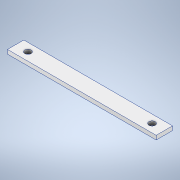
# Autodesk Inventor part: lock ring 1 supp
Saved by Autodesk Inventor 2021 (Build 250183000, 183)
## iProperties
Created: 2021-03-30
Part Number: lock ring 1 supp
Material: Aluminum 6061
Document SubType Name: Modeling
Designer: Work
Density: 2.7 g/cm^3
Appearance: Aluminum - Flat
Mass: 12.2426 g
Surface Area: 37.6973 cm^2
Volume: 4.53429 cm^3
Author: Work
Autodesk Inventor part; units mm, degrees
ref_plane "YZ Plane" through (0, 0, 0) normal (1, 0, 0) x (0, 1, 0)
ref_plane "XZ Plane" through (0, 0, 0) normal (0, 1, 0) x (-1, 0, 0)
ref_plane "XY Plane" through (0, 0, 0) normal (0, 0, 1) x (1, 0, 0)
sketch "Sketch2" plane through (0, 0, 0) normal (0, 1, 0) x (-1, 0, 0)
  line L0 (0, 0) -> (-115.5161, 0)
  line L1 (-115.5161, 0) -> (-115.5161, -12.7)
  line L2 (-115.5161, -12.7) -> (0, -12.7)
  line L3 (0, -12.7) -> (0, 0)
  line L4 (0, -6.35) -> (-115.5161, -6.35)
  point P0 (-9.525, -6.35)
  point P1 (-105.9911, -6.35)
  dimension "d12" = 12.7
  dimension "d13" = 9.525
  dimension "d14" = 9.525
  dimension "d15" = 96.4661
  constraints: 10 end point, 2 midpoint, 2 parallel, 2 point on line, 1 horizontal, 1 perpendicular
  measures "d12" distance of L2.end L0.start
  measures "d13" distance from line of L3 point (-9.525, -6.35)
  measures "d14" distance from line of L1 point (-105.991, -6.35)
  measures "d15" distance of point (-105.991, -6.35) point (-9.525, -6.35)
extrude "Extrusion2" add sketch "Sketch2" along normal blind 3.175
hole "Hole2" at (9.525, 0, -6.35) at (105.9911, 0, -6.35) direction (0, 1, 0) diameter 4.9784 end through all clearance for "Flat Head Machine Screw (82)" size "#10" standard "Ansi Unified Screw Threads"
equation "\"d15\" = ringDiam"
equation "\"height\" = 203.2"
equation "\"thickness\" = 12.7"
equation "\"shaftDiam\" = 6.35"
equation "\"shaftSpace\" = 1.5875"
equation "\"stageSpace\" = 2.54"
equation "\"stageAngle\" = 15deg"
equation "\"bearingDiam\" = 9.5504"
equation "\"FlangeDiam\" = 12.7"
equation "\"FlangeDepth\" = 1.5875"
equation "\"smallFilet\" = 0.39687"
equation "\"ringDiam\" = 96.46608"
equation "\"stockHeight\" = 50.8"
equation "\"stockWidth\" = 76.2"
equation "\"stockRad\" = 9.525"
equation "\"stockGuage\" = 3.175"
equation "\"groundActu\" = 304.8"
equation "\"baseWidth\" = 1066.8"
equation "\"baseDepth\" = 254"
equation "\"capThickness\" = 3.175"
equation "\"sup1Len\" = 660.4"
equation "\"sup1Ang\" = 22.619865deg"
equation "\"sup2Len\" = 2079.37366"
equation "\"sup2Ang\" = 8.959949deg"
equation "\"supVertLen\" = 955.13561"
equation "\"supSideLen\" = 1531.12879"
equation "\"supSideAng\" = 19.376933deg"
body "Solid2"
